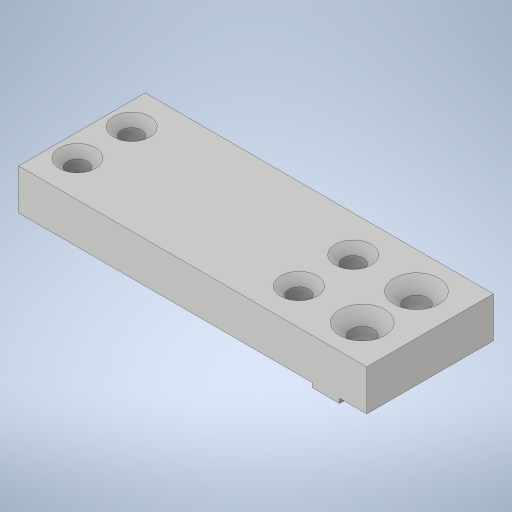
# Autodesk Inventor part: Base sujecion centelladora
Saved by Autodesk Inventor 2024.2 (Build 282272000, 272)
## iProperties
Created: 2025-06-17
Part Number: Base sujecion centelladora
Material: Genérico
Document SubType Name: Modeling
Designer: jd.castellanosq
Density: 1 g/cm^3
Appearance: Valor por defecto
Author: jd.castellanosq
Autodesk Inventor part; units mm, degrees
ref_plane "YZ Plane" through (0, 0, 0) normal (1, 0, 0) x (0, 1, 0)
ref_plane "XZ Plane" through (0, 0, 0) normal (0, 1, 0) x (-1, 0, 0)
ref_plane "XY Plane" through (0, 0, 0) normal (0, 0, 1) x (1, 0, 0)
sketch "Boceto1" plane through (0, 0, 0) normal (0, 1, 0) x (-1, 0, 0)
  line L0 (38.5, -14) -> (-38.5, -14)
  line L1 (-38.5, -14) -> (-38.5, 14)
  line L2 (-38.5, 14) -> (38.5, 14)
  line L3 (38.5, 14) -> (38.5, -14)
  circle A0 centre (-29.5, 6) radius 2.5
  circle A1 centre (-29.5, -6) radius 2.5
  point P0 (0, 0)
  point P1 (0, -14)
  point P2 (-38.5, 0)
  dimension "d0" = 5
  dimension "d1" = 9
  dimension "d2" = 77
  dimension "d3" = 28
  dimension "d17" = 8
  dimension "d18" = 5
  dimension "d19" = 12
  constraints: 8 end point, 2 centre point, 2 midpoint, 2 parallel, 2 vertical alignment, 1 horizontal, 1 horizontal alignment, 1 perpendicular
  measures "d0" diameter of A0
  measures "d1" distance from line of L1 A0.centre
  measures "d2" distance of L1.end L2.end
  measures "d3" distance of L0.end L1.end
  measures "d17" distance from line of L2 A0.centre
  measures "d18" diameter of A1
  measures "d19" distance of A0.centre A1.centre
extrude "Extrusión1" add sketch "Boceto1" along normal blind 9
sketch "Boceto2" plane through (0, 0, 0) normal (0, -1, 0) x (1, 0, 0)
  line L0 (-38.5, 14) -> (38.5, 14) projected
  line L1 (26.5, 14) -> (32.5, 14)
  line L2 (32.5, 14) -> (32.5, -14)
  line L3 (32.5, -14) -> (26.5, -14)
  line L4 (26.5, -14) -> (26.5, 14)
  line L5 (38.5, -14) -> (-38.5, -14) projected
  circle A0 centre (29.5, 6) radius 2.5 projected
  circle A1 centre (29.5, -6) radius 2.5 projected
  point P0 (0, 0)
  point P1 (29.5, 14)
  point P2 (26, 6)
  point P3 (31, 6)
  point P4 (26, -6)
  point P5 (31, -6)
  dimension "d6" = 6
  constraints: 8 end point, 2 parallel, 1 collinear, 1 horizontal, 1 midpoint, 1 perpendicular, 1 point on line, 1 vertical alignment
  measures "d6" distance between parallel lines of L2 L4
extrude "Extrusión2" add sketch "Boceto2" along normal blind 1 contours L0 L2 L3 L4 | A0 | A1
sketch "Boceto3" plane through (0, 9, 0) normal (0, 1, 0) x (1, 0, 0)
  line L0 (-38.5, 14) -> (-38.5, -14) projected
  circle A0 centre (29.5, 6) radius 2.5 projected
  circle A1 centre (29.5, -6) radius 2.5 projected
  line L1 (38.5, -14) -> (38.5, 14) projected
  line L2 (38.5, 14) -> (-38.5, 14) projected
  line L3 (-38.5, -14) -> (38.5, -14) projected
  point P0 (0, 0)
  point P1 (-33.5, 6)
  point P2 (-33.5, -6)
  point P3 (15.5, -6)
  point P4 (15.5, 6)
  dimension "d9" = 5
  dimension "d25" = 14
  constraints: 4 horizontal alignment, 2 vertical alignment
  measures "d9" distance from line of point (-33.5, 6) L0
  measures "d25" distance of A0.centre point (15.5, 6)
hole "Agujero1" at (-33.5, 9, -6) at (-33.5, 9, 6) at (15.5, 9, 6) at (15.5, 9, -6) direction (0, -1, 0) diameter 4.5 end through all countersink diameter 8 countersink angle 90 clearance for "Tornillo para maquinaria de cabeza plana" size "M4" standard "Perfil M métrico ANSI"
sketch "Boceto4" plane through (0, 9, 0) normal (0, 1, 0) x (1, 0, 0)
  circle A0 centre (29.5, 6) radius 2.5 projected
  circle A1 centre (29.5, -6) radius 2.5 projected
  point P0 (0, 0)
  constraints: 2 coincident
hole "Agujero2" at (29.5, 9, -6) at (29.5, 9, 6) direction (0, -1, 0) diameter 4.134 depth 14.2 tip angle 118 countersink diameter 10 countersink angle 90 thread size "M5x0.8" class "6H" standard "ANSI Metric M Profile"
